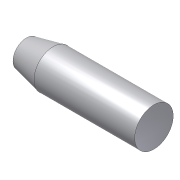
# Autodesk Inventor part: FE-00004-03
Saved by Autodesk Inventor 2012 (Build 160160000, 160)
## iProperties
Created: 2008-05-27
Part Number: FE-00004-03
Description: Connecting Pin
Document SubType Name: Modeling
Designer: narosenberg
Density: 1 g/cm^3
Mass: 119.055 g
Surface Area: 150.083 cm^2
Volume: 119.055 cm^3
Material: Default
Author: narosenberg
Autodesk Inventor part; units mm, degrees
ref_plane "YZ Plane" through (0, 0, 0) normal (1, 0, 0) x (0, 1, 0)
ref_plane "XZ Plane" through (0, 0, 0) normal (0, 1, 0) x (-1, 0, 0)
ref_plane "XY Plane" through (0, 0, 0) normal (0, 0, 1) x (1, 0, 0)
sketch "Sketch1" plane through (0, 0, 0) normal (0, 0, 1) x (1, 0, 0)
  line L0 (-63.0144, 21.5054) -> (32.2356, 21.5054)
  line L1 (32.2356, 21.5054) -> (32.2356, 3.2491)
  line L2 (32.2356, 3.2491) -> (-88.4144, 3.2491)
  line L3 (-88.4144, 3.2491) -> (-88.4144, 15.9491)
  line L4 (-88.4144, 15.9491) -> (-63.0144, 21.5054)
  dimension "d0" = 18.2563
  dimension "d1" = 25.4
  dimension "d2" = 12.7
  dimension "d3" = 120.65
  constraints: 10 end point, 2 parallel, 1 horizontal, 1 perpendicular
  measures "d0" distance of L0.end L1.end
  measures "d1" distance from line of L0.start L3
  measures "d2" distance of L2.end L3.end
  measures "d3" distance of L1.end L2.end
revolve "Revolution1" add sketch "Sketch1" angle 360 about axis through (32.2356, 3.2491, 0) along (-1, 0, 0)
body "Solid1"
